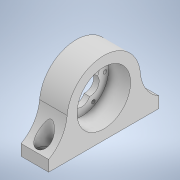
# Autodesk Inventor part: Motor Mount V2
Saved by Autodesk Inventor 2020.2 (Build 242310000, 310)
## iProperties
Created: 2020-01-13
Part Number: Motor Mount V2
Material: Generic
Document SubType Name: Modeling
Designer: maple
Density: 1 g/cm^3
Appearance: Default
Author: maple
Autodesk Inventor part; units mm, degrees
ref_plane "YZ Plane" through (0, 0, 0) normal (1, 0, 0) x (0, 1, 0)
ref_plane "XZ Plane" through (0, 0, 0) normal (0, 1, 0) x (-1, 0, 0)
ref_plane "XY Plane" through (0, 0, 0) normal (0, 0, 1) x (1, 0, 0)
sketch "Sketch1" plane through (0, 0, 0) normal (0, 1, 0) x (-1, 0, 0)
  line L0 (0, 0) -> (-19.05, 0)
  line L1 (-19.05, 0) -> (-19.05, -76.2)
  line L2 (-19.05, -76.2) -> (0, -76.2)
  line L3 (0, -76.2) -> (0, 0)
  dimension "d0" = 19.05
  dimension "d1" = 76.2
  constraints: 8 end point, 2 parallel, 1 horizontal, 1 perpendicular
  measures "d0" distance of L2.end L1.end
  measures "d1" distance of L1.end L0.end
extrude "Extrusion1" add sketch "Sketch1" along normal blind 7.62
sketch "Sketch2" plane through (0, 7.62, 0) normal (0, 1, 0) x (1, 0, 0)
  line L0 (0, 0) -> (0, 12.7)
  line L1 (0, 12.7) -> (19.05, 12.7)
  line L2 (19.05, 12.7) -> (19.05, 63.5)
  line L3 (19.05, 63.5) -> (0, 63.5)
  line L4 (0, 63.5) -> (0, 12.7)
  dimension "d4" = 12.7
  dimension "d5" = 19.05
  dimension "d6" = 50.8
  constraints: 10 end point, 2 parallel, 1 horizontal, 1 perpendicular, 1 vertical
  measures "d4" distance of L0.start L0.end
  measures "d5" distance of L3.end L2.end
  measures "d6" distance of L2.end L1.end
extrude "Extrusion2" add sketch "Sketch2" along normal blind 43.18
sketch "Sketch3" plane through (19.05, 0, 0) normal (1, 0, 0) x (0, 0, -1)
  line L0 (12.7, 50.8) -> (63.5, 50.8) projected
  line L1 (38.1, 50.8) -> (38.1, 25.4)
  circle A0 centre (38.1, 25.4) radius 18.542
  point P0 (0, 0)
  dimension "d9" = 25.4
  dimension "d10" = 37.084
  constraints: 2 end point, 1 centre point, 1 coincident, 1 midpoint, 1 vertical
  measures "d9" distance of L1.start L1.end
  measures "d10" diameter of A0
extrude "Extrusion3" cut sketch "Sketch3" against normal blind 15.24
fillet "Fillet1" radius 25.4 2 edges at (9.525, 50.8, -63.5) (9.525, 50.8, -12.7)
sketch "Sketch6" plane through (0, 7.62, 0) normal (0, 1, 0) x (1, 0, 0)
  line L0 (0, 0) -> (19.05, 0) projected
  line L1 (9.525, 0) -> (9.525, 6.35)
  line L2 (19.05, 76.2) -> (0, 76.2) projected
  line L3 (9.525, 76.2) -> (9.525, 69.85)
  dimension "d20" = 6.35
  dimension "d21" = 6.35
  constraints: 4 end point, 2 midpoint, 2 vertical
  measures "d20" distance of L1.start L1.end
  measures "d21" distance of L3.start L3.end
fillet "Fillet2" radius 25.4 2 edges at (9.525, 7.62, -63.5) (9.525, 7.62, -12.7)
hole "Hole1" at (9.525, 7.62, -6.35) at (9.525, 7.62, -69.85) direction (0, -1, 0) diameter 5.08 end through all counterbore diameter 10.16 counterbore depth 3.81
sketch "Sketch7" plane through (9.525, 7.62, -6.35) normal (0, -1, 0) x (1, 0, 0)
  circle A0 centre (0, 0) radius 5.08
  circle A1 centre (0, -63.5) radius 2.54 projected
  line L0 (-2.54, -63.5) -> (0, -63.5)
  circle A2 centre (0, -63.5) radius 5.08
  point P0 (-9.525, 6.35)
  dimension "d30" = 10.16
  dimension "d31" = 10.16
  constraints: 2 centre point, 2 end point, 1 coincident, 1 horizontal, 1 horizontal alignment, 1 other
  measures "d30" diameter of A0
  measures "d31" diameter of A2
extrude "Extrusion5" cut sketch "Sketch7" against normal blind 15.24 contours A0 | A1 | A2
sketch "Sketch10" plane through (3.81, 25.4, -38.1) normal (1, 0, 0) x (0, 0, -1)
  circle A0 centre (0, 0) radius 18.542 projected
  circle A1 centre (-8, -13.8564) radius 1.25
  circle A2 centre (0, 7) radius 6
  circle A3 centre (16, 0) radius 1.25
  circle A4 centre (8, -13.8564) radius 1.25
  circle A5 centre (-16, 0) radius 1.25
  circle A6 centre (8, -13.8564) radius 1.25
  circle A7 centre (-8, -13.8564) radius 1.25
  circle A8 centre (-8, -13.8564) radius 1.25
  circle A9 centre (-16, 0) radius 1.25
  circle A10 centre (16, 0) radius 1.25
  point P0 (-38.1, -25.4)
  constraints: 10 centre point, 4 coincident, 3 concentric
extrude "Extrusion8" cut sketch "Sketch10" against normal blind 25.4 contours A1 | A2 | A3 | A4 | A5
pattern_circular "Circular Pattern4" count 6 over 360 about axis through (19.05, 25.4, -38.1) along (-1, 0, 0) of "Extrusion8"
sketch "Sketch14" plane through (3.81, 0, 0) normal (1, 0, 0) x (0, 0, -1)
  arc A0 (36.735, 25.4) -> (37.4175, 26.5821) centre (31.9408, 28.956) ccw projected
  arc A1 (37.4175, 24.2179) -> (36.735, 25.4) centre (31.9408, 21.844) ccw projected
  arc A2 (38.7825, 24.2179) -> (37.4175, 24.2179) centre (38.1, 18.288) ccw projected
  arc A3 (39.465, 25.4) -> (38.7825, 24.2179) centre (44.2592, 21.844) ccw projected
  arc A4 (38.7825, 26.5821) -> (39.465, 25.4) centre (44.2592, 28.956) ccw projected
  arc A5 (37.4175, 26.5821) -> (38.7825, 26.5821) centre (38.1, 32.512) ccw projected
  line L0 (38.7825, 24.2179) -> (37.4175, 24.2179)
  line L1 (37.4175, 24.2179) -> (36.735, 25.4)
  line L2 (36.735, 25.4) -> (37.4175, 26.5821)
  line L3 (37.4175, 26.5821) -> (38.7825, 26.5821)
  line L4 (38.7825, 26.5821) -> (39.465, 25.4)
  line L5 (39.465, 25.4) -> (38.7825, 24.2179)
  point P0 (0, 0)
  point P1 (38.1, 25.4)
  constraints: 12 end point, 13 other
extrude "Extrusion10" cut sketch "Sketch14" against normal blind 25.4 contours A0 A5 A4 A3 A2 A1
body "Solid1"
